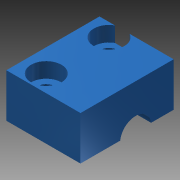
# Autodesk Inventor part: YIdlerCapLeft
Saved by Autodesk Inventor 2016 (Build 200138000, 138)
## iProperties
Category: Print
Created: 2014-08-15
Part Number: YIdlerCapLeft
Material: ABS Plastic
Document SubType Name: Modeling
Designer: t_clevj
Density: 1.06 g/cm^3
Appearance: Cyan
Mass: 4.68893 g
Surface Area: 23.1362 cm^2
Volume: 4.42352 cm^3
Vendor: Jack
Catalog Web Link: N/A
Author: t_clevj
Title: Y Idler Cap Left
Autodesk Inventor part; units mm, degrees
ref_plane "YZ Plane" through (0, 0, 0) normal (1, 0, 0) x (0, 1, 0)
ref_plane "XZ Plane" through (0, 0, 0) normal (0, 1, 0) x (-1, 0, 0)
ref_plane "XY Plane" through (0, 0, 0) normal (0, 0, 1) x (1, 0, 0)
sketch "Sketch1" plane through (0, 0, 0) normal (0, 0, 1) x (1, 0, 0)
  line L0 (0, 0) -> (19.5, 0)
  line L1 (19.5, 0) -> (19.5, 24.5)
  line L2 (19.5, 24.5) -> (0, 24.5)
  line L3 (0, 24.5) -> (0, 0)
  dimension "d0" = 24.5
  dimension "d1" = 19.5
  constraints: 8 end point, 2 parallel, 1 horizontal, 1 perpendicular
  measures "d0" distance of L2.end L0.start
  measures "d1" distance of L0.start L0.end
extrude "Extrusion1" add sketch "Sketch1" along normal blind 11.5
sketch "Sketch2" plane through (0, 0, 11.5) normal (0, 0, 1) x (1, 0, 0)
  line L0 (0, 0) -> (19.5, 0) projected
  line L1 (0, 24.5) -> (0, 0) projected
  point P0 (6, 21)
  point P1 (6, 4.5)
  dimension "d4" = 4.5
  dimension "d5" = 6
  dimension "d27" = 16.5
  constraints: 1 vertical alignment
  measures "d4" distance from line of L0 point (6, 4.5)
  measures "d5" distance from line of L1 point (6, 4.5)
  measures "d27" distance of point (6, 21) point (6, 4.5)
hole "Hole1" at (6, 21, 11.5) at (6, 4.5, 11.5) direction (0, 0, -1) diameter 4.5 end up to face face through (6.5, 16.3333, 0) facing (0, 0, -1) counterbore diameter 8 counterbore depth 4
sketch "Sketch4" plane through (0, 0, 0) normal (-1, 0, 0) x (0, 0, 1)
  line L0 (0, 24.5) -> (0, 0) projected
  line L1 (0, 24.5) -> (11.5, 24.5) projected
  circle A0 centre (-0.5, 14.5) radius 4.1
  dimension "d19" = 8.2
  dimension "d20" = 0.5
  dimension "d21" = 10
  constraints: 1 centre point
  measures "d19" diameter of A0
  measures "d20" distance from line of L0 A0.centre
  measures "d21" distance from line of L1 A0.centre
extrude "Extrusion3" cut sketch "Sketch4" against normal up to surface (19.5 mm away)
sketch "Sketch5" plane through (6, 21, 7.5) normal (0, 0, 1) x (1, 0, 0)
  circle A0 centre (0, 0) radius 4 projected
  circle A1 centre (0, -16.5) radius 3.5 projected
  circle A2 centre (0, -16.5) radius 2 projected
  point P0 (-6, -21)
body "Solid1"
